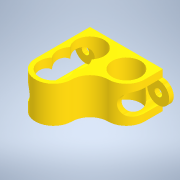
# Autodesk Inventor part: thriftybearingmount
Saved by Autodesk Inventor 2020 (Build 240168000, 168)
## iProperties
Created: 2020-03-11
Part Number: thriftybearingmount
Material: Generic
Document SubType Name: Modeling
Designer: srini
Density: 1 g/cm^3
Appearance: Glossy - Gold
Author: srini
Autodesk Inventor part; units mm, degrees
ref_plane "YZ Plane" through (0, 0, 0) normal (1, 0, 0) x (0, 1, 0)
ref_plane "XZ Plane" through (0, 0, 0) normal (0, 1, 0) x (-1, 0, 0)
ref_plane "XY Plane" through (0, 0, 0) normal (0, 0, 1) x (1, 0, 0)
sketch "Sketch1" plane through (0, 0, 0) normal (0, 0, 1) x (1, 0, 0)
  line L0 (-25.4, 12.7) -> (25.4, 12.7)
  line L1 (25.4, 12.7) -> (25.4, -12.7)
  line L2 (25.4, -12.7) -> (-25.4, -12.7)
  line L3 (-25.4, -12.7) -> (-25.4, 12.7)
  circle A0 centre (-25.4, 0) radius 7.62
  circle A1 centre (25.4, 0) radius 7.62
  point P0 (0, 0)
  point P1 (-25.4, 7.62)
  point P2 (-25.4, -7.62)
  point P3 (25.4, -7.62)
  point P4 (25.4, 7.62)
  dimension "d0" = 50.8
  dimension "d1" = 25.4
  dimension "d2" = 12.7
  dimension "d3" = 25.4
  dimension "d4" = 15.24
  constraints: 8 end point, 2 centre point, 2 midpoint, 2 parallel, 1 equal radius, 1 horizontal, 1 perpendicular
  measures "d0" distance of L0.start L0.end
  measures "d1" distance of L2.end L0.start
  measures "d2" distance from line of point (0, 0) L0
  measures "d3" distance from line of point (0, 0) L3
  measures "d4" diameter of A0
extrude "Extrusion1" add sketch "Sketch1" along normal blind 3.175
sketch "Sketch2" plane through (0, 0, 3.175) normal (0, 0, 1) x (1, 0, 0)
  line L0 (25.4, -12.7) -> (25.4, -7.62) projected
  arc A0 (25.4, -7.62) -> (25.4, 7.62) centre (25.4, 0) ccw projected
  line L1 (25.4, 7.62) -> (25.4, 12.7) projected
  line L2 (25.4, 12.7) -> (-25.4, 12.7) projected
  line L3 (-25.4, 12.7) -> (-25.4, 7.62) projected
  arc A1 (-25.4, 7.62) -> (-25.4, -7.62) centre (-25.4, 0) ccw projected
  line L4 (-25.4, -7.62) -> (-25.4, -12.7) projected
  line L5 (-25.4, -12.7) -> (25.4, -12.7) projected
  circle A2 centre (-25.4, 0) radius 7.62
  line L6 (25.4, 7.62) -> (25.4, 12.7) projected
  circle A3 centre (25.4, 0) radius 7.62
  point P0 (0, 0)
  constraints: 2 coincident, 6 other
extrude "Extrusion2" add sketch "Sketch2" along normal blind 22.225 contours L5 L4 A2 L3 L2 L1 A3 L0
sketch "Sketch4" plane through (0, 0, 25.4) normal (0, 0, 1) x (1, 0, 0)
  line L0 (-25.4, 12.7) -> (-25.4, 7.62) projected
  arc A0 (-25.4, -7.62) -> (-25.4, 7.62) centre (-25.4, 0) ccw projected
  line L1 (-25.4, -7.62) -> (-25.4, -12.7) projected
  line L2 (-25.4, -12.7) -> (25.4, -12.7) projected
  line L3 (25.4, -12.7) -> (25.4, -7.62) projected
  arc A1 (25.4, 7.62) -> (25.4, -7.62) centre (25.4, 0) ccw projected
  line L4 (25.4, 7.62) -> (25.4, 12.7) projected
  line L5 (25.4, 12.7) -> (-25.4, 12.7) projected
  line L6 (0, 12.7) -> (0, -12.7)
  point P0 (0, 0)
  constraints: 2 end point, 2 midpoint
extrude "Extrusion3" add sketch "Sketch4" along normal blind 25.4 contours L5 L6 L2 L1 A0 L0
sketch "Sketch5" plane through (-25.4, 12.7, 0) normal (0, 1, 0) x (1, 0, 0)
  circle A0 centre (12.7, -38.1) radius 9.825
  line L0 (0, 0) -> (0, -50.8) projected
  line L1 (50.8, 0) -> (0, 0) projected
  circle A1 centre (12.7, -25.4) radius 9.825
  circle A2 centre (12.7, -12.7) radius 9.825
  circle A3 centre (38.1, -38.1) radius 9.825
  circle A4 centre (38.1, -25.4) radius 9.825
  circle A5 centre (38.1, -12.7) radius 9.825
  point P0 (25.4, 0)
  point P1 (5.2028, -31.75)
  point P2 (20.1972, -31.75)
  point P3 (20.1972, -19.05)
  point P4 (5.2028, -19.05)
  dimension "d11" = 19.65
  dimension "d12" = 12.7
  dimension "d13" = 38.1
  dimension "d16" = 12.7
  dimension "d19" = 25.4
  constraints: 6 centre point, 1 horizontal, 1 vertical, 10 other
  measures "d11" diameter of A0
  measures "d12" distance from line of A0.centre L0
  measures "d13" distance from line of A0.centre L1
  measures "d16" distance of A0.centre A1.centre
  measures "d19" distance of A0.centre A3.centre
extrude "Extrusion4" cut sketch "Sketch5" against normal through all contours A0 A1 | A1 A0 | A0 A1 A2 | A2 A1 | A1 A2 | A3 A4 | A4 A3 | A5 A4 | A4 A5
sketch "Sketch6" plane through (0, 0, 0) normal (0, 0, -1) x (-1, 0, 0)
  circle A0 centre (-25.4, 0) radius 2.5781
  circle A1 centre (25.4, 0) radius 2.5781
  arc A2 (-25.4, 7.62) -> (-25.4, -7.62) centre (-25.4, 0) ccw projected
  arc A3 (25.4, -7.62) -> (25.4, 7.62) centre (25.4, 0) ccw projected
  point P0 (0, 0)
  dimension "d24" = 5.1562
  constraints: 2 centre point, 2 concentric, 1 equal radius
  measures "d24" diameter of A0
extrude "Extrusion5" cut sketch "Sketch6" against normal through all
fillet "Fillet1" radius 12.7 6 edges at (-25.4, 10.16, 50.8) (-25.4, -10.16, 50.8) (0, 0, 50.8) (0, 0, 25.4) (25.4, -10.16, 25.4) (25.4, 10.16, 25.4)
equation "\"d2\" = 0.5 * d1"
equation "\"d3\" = 0.5 * d0"
body "Solid1"
